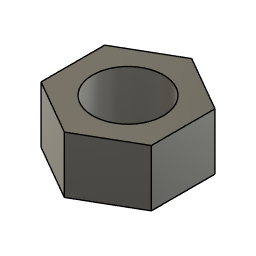
M5 nut v1 (Autodesk Fusion 360 design; units mm, degrees)
Autodesk Fusion 360 part; units mm, degrees
sketch "Sketch1" plane through (0, 0, 0) normal (0, 1, 0) x (1, 0, 0)
  line L0 (-3.9, -2.2517) -> (0, -4.5033)
  line L1 (0, -4.5033) -> (3.9, -2.2517)
  line L2 (3.9, -2.2517) -> (3.9, 2.2517)
  line L3 (3.9, 2.2517) -> (0, 4.5033)
  line L4 (0, 4.5033) -> (-3.9, 2.2517)
  line L5 (-3.9, 2.2517) -> (-3.9, -2.2517)
  circle A0 centre (0, 0) radius 2.5
  dimension "d2" = 7.8
  dimension "d3" = 5
  constraint coincident A0.centre origin
  measures "d2" distance of L2 L5
  measures "d3" diameter of A0
extrude "Extrude1" add sketch "Sketch1" along normal blind 4
